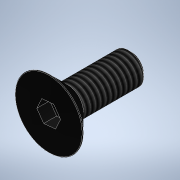
# Autodesk Inventor part: SCREW,FLAT HD,P,12.9,M6X1.00X16MM
Saved by Autodesk Inventor 2022.4 (Build 264492000, 492)
## iProperties
Manager: 100-07253
Shininess: 64.0
Length Units: 11269
Angle Units: 11279
Time Units: 11290
Mass Units: 11283
Length Display Precision: 3
Angle Display Precision: 2
Created: 2021-07-09
Part Number: SCREW,FLAT HD,P,12.9,M6X1.00X16MM
Material: Default
Document SubType Name: Modeling
Designer: cdotson
Description: SCREW, FLAT HD, P, 12_9, M6X1_00X16MM
Density: 1 g/cm^3
Appearance: Glossy - Black
Mfg Approved By: Cathy.Lesperance
Mass: 0.5984 g
Surface Area: 5.79435 cm^2
Volume: 0.5984 cm^3
Engr Approved By: P
Checked By: 0003189965
User Status: Released
Density: 0.0
Volumn: 0.0
Area: 0.0
PropertySet Name: Model Information
Control State: 0
Master: False
Checked Out: False
CN_MASS: 0.0
ModelCat: Uncategorized
FIRST_DESCRIPTION: _
SECOND_DESCRIPTION: _
THIRD_DESCRIPTION: _
CN_SERVICEABLE: _
PTC_WM_ITERATION: 3
PTC_WM_ORGANIZATION_ID: CLWC
PTC_WM_LIFECYCLE: CLWC_CAD_LC
Author: -
Subject: -
Keywords: -
Revision Number: A
Autodesk Inventor part; units mm, degrees
ref_plane "YZ Plane" through (0, 0, 0) normal (1, 0, 0) x (0, 1, 0)
ref_plane "XZ Plane" through (0, 0, 0) normal (0, 1, 0) x (-1, 0, 0)
ref_plane "XY Plane" through (0, 0, 0) normal (0, 0, 1) x (1, 0, 0)
sketch "Sketch1" plane through (0, 0, 0) normal (0, 0, 1) x (1, 0, 0)
  circle A0 centre (0, 0) radius 3
  dimension "Diameter" = 6
  constraints: 1 centre point
  measures "Diameter" diameter of A0
extrude "Extrusion1" add sketch "Sketch1" along normal blind 12.28
sketch "Sketch2" plane through (0, 0, 12.28) normal (0, 0, 1) x (1, 0, 0)
  circle A0 centre (0, 0) radius 3 projected
extrude "Extrusion2" add sketch "Sketch2" along normal blind 3.72 draft 45
sketch "Sketch3" plane through (0, 0, 16) normal (0, 0, 1) x (1, 0, 0)
  circle A0 centre (0, 0) radius 6.72 projected
  circle A1 centre (0, 0) radius 2.3094 construction
  line L0 (0.9667, 2.0973) -> (2.2997, 0.2115)
  line L1 (2.2997, 0.2115) -> (1.333, -1.8859)
  line L2 (1.333, -1.8859) -> (-0.9667, -2.0973)
  line L3 (-0.9667, -2.0973) -> (-2.2997, -0.2115)
  line L4 (-2.2997, -0.2115) -> (-1.333, 1.8859)
  line L5 (-1.333, 1.8859) -> (0.9667, 2.0973)
  dimension "Hex_Width" = 4
  constraints: 12 end point, 6 point on circle, 4 equal length, 1 centre point, 1 coincident
  measures "Hex_Width" distance between parallel lines of L0 L3
extrude "Extrusion3" cut sketch "Sketch3" against normal blind 2.5 contours L0 L1 L2 L3 L4 L5
thread "Thread1" size "M6x1" class "4g6g" standard "ANSI Metric M Profile" length 12.28
chamfer "Chamfer2" distance 0.6 angle 45 1 edges at (-3, 0, 0)
fillet "Fillet1" radius 0.1 1 edges at (-6.72, 0, 16)
equation "\"d10\" = Thread_Length"
equation "\"d13\" = Chamfer"
equation "\"Thread_Length\" = 12.28"
equation "\"Length\" = 16"
equation "\"Chamfer\" = 0.6"
body "Solid1"
